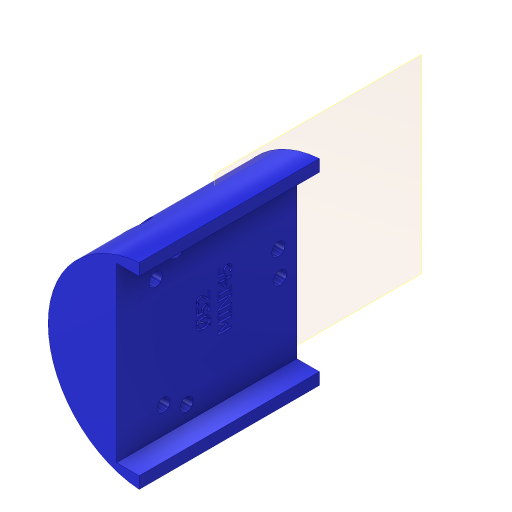
# Autodesk Inventor part: MINI45NewShell52v2-1_B
Saved by Autodesk Inventor 2023 (Build 270158000, 158)
## iProperties
Created: 2016-07-01
Part Number: MINI45NewShell52v2-1_B
Material: ABS Plastic
Document SubType Name: Modeling
Designer: Administrateur
Density: 1.06 g/cm^3
Appearance: Blue - Wall Paint - Glossy
Author: Administrateur
Autodesk Inventor part; units mm, degrees
ref_plane "XZ Plane" through (0, 0, 0) normal (0, 1, 0) x (-1, 0, 0)
sketch "Sketch1" plane through (0, 0, 0) normal (0, 0, 1) x (1, 0, 0)
  arc A0 (0, 26.2509) -> (0, -26.2509) centre (0, 0) ccw
  line L0 (0, 26.2509) -> (0, 23)
  line L1 (0, 23) -> (-8, 23)
  line L2 (-8, 23) -> (-8, 0)
  line L3 (-46.5484, 0) -> (26.4312, 0) construction
  line L4 (0, -26.2509) -> (0, -23)
  line L5 (0, -23) -> (-8, -23)
  line L6 (-8, -23) -> (-8, 0)
  dimension "d2" = 26.2509
  dimension "d3" = 46
  dimension "d4" = 8
  dimension "d27" = 23
  dimension "d28" = 3.2509
  constraints: 14 end point, 2 horizontal, 2 point on circle, 2 symmetric about line, 1 centre point, 1 coincident, 1 perpendicular, 1 vertical
  measures "d2" radius of A0
  measures "d3" distance between parallel lines of L5 L1
  measures "d4" distance of L0.end L1.end
  measures "d27" distance of L1.end L2.end
  measures "d28" distance of L0.start L0.end
extrude "Extrusion1" add sketch "Sketch1" along normal blind 120
sketch "Sketch2" plane through (-8, -23, 0) normal (1, 0, 0) x (0, 0, -1)
  line L0 (-60, 23) -> (-120, 23) construction
  line L1 (-120, 49.2509) -> (-120, -3.2509) construction
  line L2 (0, 49.2509) -> (-120, 49.2509) construction
  line L3 (-60, 49.2509) -> (-60, -3.2509) construction
  line L4 (0, -3.2509) -> (-120, -3.2509) construction
  line L5 (-60, 23) -> (-73.6292, 37.1134) construction
  circle A0 centre (-60, 23) radius 19.62 construction
  line L6 (-60, 23) -> (-67.9802, 40.9238) construction
  line L7 (-60, 23) -> (-65.408, 4.14) construction
  line L8 (-60, 23) -> (-71.5323, 7.1271) construction
  line L9 (-60, 23) -> (-40.9628, 27.7465) construction
  line L10 (-60, 23) -> (-40.4875, 20.9492) construction
  point P0 (0, 23)
  dimension "d32" = 39.24
  dimension "d34" = 20
  dimension "d37" = 360
  dimension "d39" = 66
  constraints: 16 end point, 11 coincident, 4 midpoint, 2 point on circle, 1 centre point, 17 other
  measures "d32" diameter of A0
  measures "d34" angle of L5 L6
  measures "d39" angle of L0 L6
hole "Hole1" at (-8, 17.9238, 67.9802) at (-8, 14.1134, 73.6292) at (-8, -15.8729, 71.5323) at (-8, -18.86, 65.408) at (-8, -2.0508, 40.4875) at (-8, 4.7465, 40.9628) direction (-1, 0, 0) diameter 3.5 end through all
ref_plane "Work Plane1" through (-26.2509, 0, 0) normal (1, 0, 0) x (0, 1, 0)
ref_plane "Work Plane2" through (-10, 0, 0) normal (1, 0, 0) x (0, 1, 0)
ref_plane "Work Plane3" through (-13.3, -23, 0) normal (1, 0, 0) x (0, 0, -1)
sketch "Sketch4" plane through (-13.3, -23, 0) normal (1, 0, 0) x (0, 0, -1)
  line L0 (0, 49.2509) -> (0, -3.2509) projected
  line L1 (0, -3.2509) -> (-120, -3.2509) projected
  line L2 (-120, 49.2509) -> (-120, -3.2509) projected
  line L3 (0, 49.2509) -> (-120, 49.2509) projected
  circle A0 centre (-67.9802, 40.9238) radius 1.75 projected
  circle A1 centre (-73.6292, 37.1134) radius 1.75 projected
  circle A2 centre (-71.5323, 7.1271) radius 1.75 projected
  circle A3 centre (-65.408, 4.14) radius 1.75 projected
  circle A4 centre (-40.4875, 20.9492) radius 1.75 projected
  circle A5 centre (-40.9628, 27.7465) radius 1.75 projected
  point P0 (0, 23)
  point P1 (-40.4875, 22.6992)
  point P2 (-71.5323, 8.8771)
  point P3 (-67.9802, 42.6738)
  point P4 (-73.6292, 38.8634)
  point P5 (-65.408, 5.89)
  point P6 (-40.9628, 29.4965)
  constraints: 6 coincident, 6 vertical alignment, 6 other
hole "Hole3" at (-13.3, 17.9238, 67.9802) at (-13.3, 14.1134, 73.6292) at (-13.3, -15.8729, 71.5323) at (-13.3, -18.86, 65.408) at (-13.3, -2.0508, 40.4875) at (-13.3, 4.7465, 40.9628) direction (-1, 0, 0) diameter 6.5 end through all
sketch "Sketch5" plane through (-8, -23, 0) normal (1, 0, 0) x (0, 0, -1)
  line L0 (-62.902, 19.0607) -> (-62.902, 27.7199) construction
  line L1 (-62.902, 27.7199) -> (-58.9141, 27.7199) construction
  line L2 (-58.9141, 27.7199) -> (-58.9141, 19.0607) construction
  line L3 (-58.9141, 19.0607) -> (-62.902, 19.0607) construction
  spline S0 degree 2 poles (-60.9364, 22.3111) (-60.0685, 22.3111) (-59.1127, 21.4659) (-59.1127, 20.7625) knots 0 0 0 1 2 2 2
  spline S1 degree 2 poles (-59.1127, 20.7625) (-59.1127, 20.5044) (-59.2488, 20.0591) (-59.3736, 19.8804) knots 0 0 0 1 2 2 2
  line L4 (-59.3736, 19.8804) -> (-58.9141, 19.5684)
  line L5 (-58.9141, 19.5684) -> (-58.9141, 19.2224)
  line L6 (-58.9141, 19.2224) -> (-59.5665, 19.6648)
  spline S2 degree 2 poles (-59.5665, 19.6648) (-59.7991, 19.4549) (-60.4855, 19.2167) (-60.9364, 19.2167) knots 0 0 0 1 2 2 2
  spline S3 degree 2 poles (-60.9364, 19.2167) (-61.8015, 19.2167) (-62.7602, 20.0647) (-62.7602, 20.7625) knots 0 0 0 1 2 2 2
  spline S4 degree 2 poles (-62.7602, 20.7625) (-62.7602, 21.0319) (-62.6297, 21.4517) (-62.5021, 21.6389) knots 0 0 0 1 2 2 2
  line L7 (-62.5021, 21.6389) -> (-62.902, 21.9083)
  line L8 (-62.902, 21.9083) -> (-62.902, 22.2572)
  line L9 (-62.902, 22.2572) -> (-62.312, 21.8544)
  spline S5 degree 2 poles (-62.312, 21.8544) (-62.0795, 22.07) (-61.4044, 22.3111) (-60.9364, 22.3111) knots 0 0 0 1 2 2 2
  spline S6 degree 2 poles (-60.9364, 21.8318) (-61.2598, 21.8318) (-61.7675, 21.7013) (-61.9348, 21.5935) knots 0 0 0 1 2 2 2
  line L10 (-61.9348, 21.5935) -> (-59.731, 20.1186)
  spline S7 degree 2 poles (-59.731, 20.1186) (-59.6232, 20.2519) (-59.5154, 20.5526) (-59.5154, 20.7653) knots 0 0 0 1 2 2 2
  spline S8 degree 2 poles (-59.5154, 20.7653) (-59.5154, 21.2503) (-60.2472, 21.8318) (-60.9364, 21.8318) knots 0 0 0 1 2 2 2
  spline S9 degree 2 poles (-62.1475, 21.4006) (-62.2525, 21.2787) (-62.3574, 20.9582) (-62.3574, 20.7653) knots 0 0 0 1 2 2 2
  spline S10 degree 2 poles (-62.3574, 20.7653) (-62.3574, 20.2775) (-61.6342, 19.696) (-60.9364, 19.696) knots 0 0 0 1 2 2 2
  spline S11 degree 2 poles (-60.9364, 19.696) (-60.6188, 19.696) (-60.1252, 19.818) (-59.9494, 19.9286) knots 0 0 0 1 2 2 2
  line L11 (-59.9494, 19.9286) -> (-62.1475, 21.4006)
  spline S12 degree 2 poles (-60.2983, 24.8439) (-60.0458, 24.8439) (-59.6147, 24.6822) (-59.4559, 24.5348) knots 0 0 0 1 2 2 2
  spline S13 degree 2 poles (-59.4559, 24.5348) (-59.297, 24.3873) (-59.1127, 23.9476) (-59.1127, 23.6754) knots 0 0 0 1 2 2 2
  spline S14 degree 2 poles (-59.1127, 23.6754) (-59.1127, 23.4258) (-59.2233, 22.9379) (-59.3112, 22.7592) knots 0 0 0 1 2 2 2
  line L12 (-59.3112, 22.7592) -> (-59.8076, 22.7592)
  line L13 (-59.8076, 22.7592) -> (-59.8076, 22.7933)
  spline S15 degree 2 poles (-59.8076, 22.7933) (-59.7679, 22.8472) (-59.6658, 23.0485) (-59.6204, 23.1705) knots 0 0 0 1 2 2 2
  spline S16 degree 2 poles (-59.6204, 23.1705) (-59.5722, 23.3095) (-59.5183, 23.5392) (-59.5183, 23.6839) knots 0 0 0 1 2 2 2
  spline S17 degree 2 poles (-59.5183, 23.6839) (-59.5183, 23.8257) (-59.6204, 24.0923) (-59.731, 24.1887) knots 0 0 0 1 2 2 2
  spline S18 degree 2 poles (-59.731, 24.1887) (-59.8359, 24.2766) (-60.1139, 24.3674) (-60.3011, 24.3674) knots 0 0 0 1 2 2 2
  spline S19 degree 2 poles (-60.3011, 24.3674) (-60.4883, 24.3674) (-60.7265, 24.2653) (-60.806, 24.1689) knots 0 0 0 1 2 2 2
  spline S20 degree 2 poles (-60.806, 24.1689) (-60.8939, 24.0696) (-60.9676, 23.7746) (-60.9676, 23.5959) knots 0 0 0 1 2 2 2
  spline S21 degree 2 poles (-60.9676, 23.5959) (-60.9676, 23.4031) (-60.9081, 23.0202) (-60.8825, 22.9039) knots 0 0 0 1 2 2 2
  line L14 (-60.8825, 22.9039) -> (-62.6864, 22.9039)
  line L15 (-62.6864, 22.9039) -> (-62.6864, 24.8241)
  line L16 (-62.6864, 24.8241) -> (-62.2752, 24.8241)
  line L17 (-62.2752, 24.8241) -> (-62.2752, 23.3549)
  line L18 (-62.2752, 23.3549) -> (-61.342, 23.3549)
  spline S22 degree 2 poles (-61.342, 23.3549) (-61.3534, 23.4399) (-61.3619, 23.6044) (-61.3619, 23.6725) knots 0 0 0 1 2 2 2
  spline S23 degree 2 poles (-61.3619, 23.6725) (-61.3619, 23.942) (-61.274, 24.3135) (-61.1435, 24.4837) knots 0 0 0 1 2 2 2
  spline S24 degree 2 poles (-61.1435, 24.4837) (-61.013, 24.6567) (-60.6159, 24.8439) (-60.2983, 24.8439) knots 0 0 0 1 2 2 2
  line L19 (-59.1864, 27.5072) -> (-59.1864, 25.3488)
  line L20 (-59.1864, 25.3488) -> (-59.6828, 25.3488)
  spline S25 degree 2 poles (-59.6828, 25.3488) (-59.9012, 25.5813) (-60.3068, 25.9955) (-60.5252, 26.194) knots 0 0 0 1 2 2 2
  spline S26 degree 2 poles (-60.5252, 26.194) (-60.9648, 26.5939) (-61.4923, 26.886) (-61.7731, 26.886) knots 0 0 0 1 2 2 2
  spline S27 degree 2 poles (-61.7731, 26.886) (-61.9206, 26.886) (-62.1419, 26.7953) (-62.2128, 26.713) knots 0 0 0 1 2 2 2
  spline S28 degree 2 poles (-62.2128, 26.713) (-62.2837, 26.6308) (-62.3546, 26.4152) (-62.3546, 26.2848) knots 0 0 0 1 2 2 2
  spline S29 degree 2 poles (-62.3546, 26.2848) (-62.3546, 26.16) (-62.2922, 25.9047) (-62.244, 25.7884) knots 0 0 0 1 2 2 2
  spline S30 degree 2 poles (-62.244, 25.7884) (-62.2043, 25.6891) (-62.0908, 25.5048) (-62.0511, 25.448) knots 0 0 0 1 2 2 2
  line L21 (-62.0511, 25.448) -> (-62.0511, 25.4225)
  line L22 (-62.0511, 25.4225) -> (-62.5503, 25.4225)
  spline S31 degree 2 poles (-62.5503, 25.4225) (-62.6212, 25.5672) (-62.7602, 26.0862) (-62.7602, 26.3188) knots 0 0 0 1 2 2 2
  spline S32 degree 2 poles (-62.7602, 26.3188) (-62.7602, 26.8095) (-62.2411, 27.3625) (-61.7987, 27.3625) knots 0 0 0 1 2 2 2
  spline S33 degree 2 poles (-61.7987, 27.3625) (-61.5916, 27.3625) (-61.2456, 27.2661) (-61.0981, 27.181) knots 0 0 0 1 2 2 2
  spline S34 degree 2 poles (-61.0981, 27.181) (-60.9449, 27.0959) (-60.6443, 26.8492) (-60.4996, 26.713) knots 0 0 0 1 2 2 2
  spline S35 degree 2 poles (-60.4996, 26.713) (-60.2586, 26.4918) (-59.7423, 25.9501) (-59.592, 25.7884) knots 0 0 0 1 2 2 2
  line L23 (-59.592, 25.7884) -> (-59.592, 27.5072)
  line L24 (-59.592, 27.5072) -> (-59.1864, 27.5072)
  line L25 (-53.4238, 18.8621) -> (-53.4238, 18.397)
  line L26 (-53.4238, 18.397) -> (-56.4388, 18.397)
  line L27 (-56.4388, 18.397) -> (-54.3881, 17.4837)
  line L28 (-54.3881, 17.4837) -> (-54.3881, 17.2001)
  line L29 (-54.3881, 17.2001) -> (-56.4388, 16.2953)
  line L30 (-56.4388, 16.2953) -> (-53.4238, 16.2953)
  line L31 (-53.4238, 16.2953) -> (-53.4238, 15.8613)
  line L32 (-53.4238, 15.8613) -> (-56.9238, 15.8613)
  line L33 (-56.9238, 15.8613) -> (-56.9238, 16.4967)
  line L34 (-56.9238, 16.4967) -> (-54.9752, 17.3702)
  line L35 (-54.9752, 17.3702) -> (-56.9238, 18.2155)
  line L36 (-56.9238, 18.2155) -> (-56.9238, 18.8621)
  line L37 (-56.9238, 18.8621) -> (-53.4238, 18.8621)
  line L38 (-53.4238, 20.7908) -> (-53.4238, 19.4351)
  line L39 (-53.4238, 19.4351) -> (-53.7811, 19.4351)
  line L40 (-53.7811, 19.4351) -> (-53.7811, 19.8804)
  line L41 (-53.7811, 19.8804) -> (-56.5664, 19.8804)
  line L42 (-56.5664, 19.8804) -> (-56.5664, 19.4351)
  line L43 (-56.5664, 19.4351) -> (-56.9238, 19.4351)
  line L44 (-56.9238, 19.4351) -> (-56.9238, 20.7908)
  line L45 (-56.9238, 20.7908) -> (-56.5664, 20.7908)
  line L46 (-56.5664, 20.7908) -> (-56.5664, 20.3455)
  line L47 (-56.5664, 20.3455) -> (-53.7811, 20.3455)
  line L48 (-53.7811, 20.3455) -> (-53.7811, 20.7908)
  line L49 (-53.7811, 20.7908) -> (-53.4238, 20.7908)
  line L50 (-53.4238, 23.8711) -> (-53.4238, 23.3492)
  line L51 (-53.4238, 23.3492) -> (-56.4416, 21.8006)
  line L52 (-56.4416, 21.8006) -> (-53.4238, 21.8006)
  line L53 (-53.4238, 21.8006) -> (-53.4238, 21.3666)
  line L54 (-53.4238, 21.3666) -> (-56.9238, 21.3666)
  line L55 (-56.9238, 21.3666) -> (-56.9238, 22.0275)
  line L56 (-56.9238, 22.0275) -> (-54.1527, 23.4371)
  line L57 (-54.1527, 23.4371) -> (-56.9238, 23.4371)
  line L58 (-56.9238, 23.4371) -> (-56.9238, 23.8711)
  line L59 (-56.9238, 23.8711) -> (-53.4238, 23.8711)
  line L60 (-53.4238, 25.7997) -> (-53.4238, 24.444)
  line L61 (-53.4238, 24.444) -> (-53.7811, 24.444)
  line L62 (-53.7811, 24.444) -> (-53.7811, 24.8893)
  line L63 (-53.7811, 24.8893) -> (-56.5664, 24.8893)
  line L64 (-56.5664, 24.8893) -> (-56.5664, 24.444)
  line L65 (-56.5664, 24.444) -> (-56.9238, 24.444)
  line L66 (-56.9238, 24.444) -> (-56.9238, 25.7997)
  line L67 (-56.9238, 25.7997) -> (-56.5664, 25.7997)
  line L68 (-56.5664, 25.7997) -> (-56.5664, 25.3544)
  line L69 (-56.5664, 25.3544) -> (-53.7811, 25.3544)
  line L70 (-53.7811, 25.3544) -> (-53.7811, 25.7997)
  line L71 (-53.7811, 25.7997) -> (-53.4238, 25.7997)
  line L72 (-54.6264, 28.5283) -> (-54.6264, 28.1113)
  line L73 (-54.6264, 28.1113) -> (-53.4238, 28.1113)
  line L74 (-53.4238, 28.1113) -> (-53.4238, 27.6604)
  line L75 (-53.4238, 27.6604) -> (-54.6264, 27.6604)
  line L76 (-54.6264, 27.6604) -> (-54.6264, 26.1146)
  line L77 (-54.6264, 26.1146) -> (-55.1199, 26.1146)
  line L78 (-55.1199, 26.1146) -> (-56.9238, 27.6802)
  line L79 (-56.9238, 27.6802) -> (-56.9238, 28.1113)
  line L80 (-56.9238, 28.1113) -> (-55.0036, 28.1113)
  line L81 (-55.0036, 28.1113) -> (-55.0036, 28.5283)
  line L82 (-55.0036, 28.5283) -> (-54.6264, 28.5283)
  line L83 (-55.0036, 27.6604) -> (-56.3707, 27.6604)
  line L84 (-56.3707, 27.6604) -> (-55.0036, 26.4833)
  line L85 (-55.0036, 26.4833) -> (-55.0036, 27.6604)
  spline S36 degree 2 poles (-54.5356, 31.0242) (-54.2832, 31.0242) (-53.8521, 30.8625) (-53.6932, 30.7151) knots 0 0 0 1 2 2 2
  spline S37 degree 2 poles (-53.6932, 30.7151) (-53.5344, 30.5676) (-53.35, 30.1279) (-53.35, 29.8557) knots 0 0 0 1 2 2 2
  spline S38 degree 2 poles (-53.35, 29.8557) (-53.35, 29.6061) (-53.4606, 29.1182) (-53.5486, 28.9395) knots 0 0 0 1 2 2 2
  line L86 (-53.5486, 28.9395) -> (-54.0449, 28.9395)
  line L87 (-54.0449, 28.9395) -> (-54.0449, 28.9736)
  spline S39 degree 2 poles (-54.0449, 28.9736) (-54.0052, 29.0275) (-53.9031, 29.2288) (-53.8577, 29.3508) knots 0 0 0 1 2 2 2
  spline S40 degree 2 poles (-53.8577, 29.3508) (-53.8095, 29.4898) (-53.7556, 29.7195) (-53.7556, 29.8642) knots 0 0 0 1 2 2 2
  spline S41 degree 2 poles (-53.7556, 29.8642) (-53.7556, 30.006) (-53.8577, 30.2726) (-53.9683, 30.369) knots 0 0 0 1 2 2 2
  spline S42 degree 2 poles (-53.9683, 30.369) (-54.0733, 30.457) (-54.3512, 30.5477) (-54.5384, 30.5477) knots 0 0 0 1 2 2 2
  spline S43 degree 2 poles (-54.5384, 30.5477) (-54.7256, 30.5477) (-54.9639, 30.4456) (-55.0433, 30.3492) knots 0 0 0 1 2 2 2
  spline S44 degree 2 poles (-55.0433, 30.3492) (-55.1312, 30.2499) (-55.205, 29.9549) (-55.205, 29.7762) knots 0 0 0 1 2 2 2
  spline S45 degree 2 poles (-55.205, 29.7762) (-55.205, 29.5834) (-55.1454, 29.2005) (-55.1199, 29.0842) knots 0 0 0 1 2 2 2
  line L88 (-55.1199, 29.0842) -> (-56.9238, 29.0842)
  line L89 (-56.9238, 29.0842) -> (-56.9238, 31.0044)
  line L90 (-56.9238, 31.0044) -> (-56.5125, 31.0044)
  line L91 (-56.5125, 31.0044) -> (-56.5125, 29.5352)
  line L92 (-56.5125, 29.5352) -> (-55.5794, 29.5352)
  spline S46 degree 2 poles (-55.5794, 29.5352) (-55.5907, 29.6202) (-55.5992, 29.7848) (-55.5992, 29.8528) knots 0 0 0 1 2 2 2
  spline S47 degree 2 poles (-55.5992, 29.8528) (-55.5992, 30.1223) (-55.5113, 30.4938) (-55.3808, 30.664) knots 0 0 0 1 2 2 2
  spline S48 degree 2 poles (-55.3808, 30.664) (-55.2504, 30.837) (-54.8533, 31.0242) (-54.5356, 31.0242) knots 0 0 0 1 2 2 2
  point P0 (0, 23)
  constraints: 2 other
extrude "Extrusion2" cut sketch "Sketch5" against normal blind 2
sketch "Sketch6" plane through (-8, -23, 0) normal (1, 0, 0) x (0, 0, -1)
  line L0 (-120, 49.2509) -> (-120, -3.2509) projected
  line L1 (0, -3.2509) -> (-120, -3.2509) projected
  line L2 (-120, 49.2509) -> (-84, 49.2509)
  line L3 (-84, 49.2509) -> (-84, -3.2509)
  line L4 (-84, -3.2509) -> (-120, -3.2509)
  line L5 (-120, -3.2509) -> (-120, 49.2509)
  line L6 (0, 49.2509) -> (0, -3.2509) projected
  line L7 (0, 49.2509) -> (-36, 49.2509)
  line L8 (-36, 49.2509) -> (-36, -3.2509)
  line L9 (-36, -3.2509) -> (0, -3.2509)
  line L10 (0, -3.2509) -> (0, 49.2509)
  line L11 (0, 49.2509) -> (-120, 49.2509) construction
  line L12 (-60, 49.2509) -> (-60, -34.7766) construction
  point P0 (0, 23)
  point P1 (-36, -3.2509)
  dimension "d50" = 24
  dimension "d51" = 24
  constraints: 18 end point, 4 parallel, 2 horizontal, 2 perpendicular, 2 point on line, 1 midpoint, 1 vertical
  measures "d50" distance between parallel lines of L3 L12
  measures "d51" distance between parallel lines of L8 L12
extrude "Extrusion3" cut sketch "Sketch6" along normal through all both and the other way through all
sketch "Sketch7" plane through (0, 23, 36) normal (1, 0, 0) x (0, 0, -1)
  line L0 (0, 0) -> (0, 3.2509) projected
  line L1 (0, 3.2509) -> (-48, 3.2509) projected
  line L2 (-48, 3.2509) -> (-48, 0) projected
  line L3 (0, 0) -> (-48, 0) projected
  line L4 (0, -49.2509) -> (0, -46) projected
  line L5 (0, -46) -> (-48, -46) projected
  line L6 (-48, -46) -> (-48, -49.2509) projected
  line L7 (0, -49.2509) -> (-48, -49.2509) projected
  point P0 (36, -23)
extrude "Extrusion4" cut sketch "Sketch7" against normal blind 2
equation "\"d27\" = 0.5 * d3"
equation "\"d28\" = -0.5 * d3 + d2"
equation "\"d51\" = d50"
body "Solid1"
